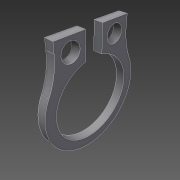
# Autodesk Inventor part: Horseshoe Clip
Saved by Autodesk Inventor 2016 (Build 200138000, 138)
## iProperties
Created: 2012-08-29
Part Number: Horseshoe Clip
Material: Generic
Document SubType Name: Modeling
Designer: John
Density: 1 g/cm^3
Appearance: Default
Author: John
Autodesk Inventor part; units mm, degrees
ref_plane "YZ Plane" through (0, 0, 0) normal (1, 0, 0) x (0, 1, 0)
ref_plane "XZ Plane" through (0, 0, 0) normal (0, 1, 0) x (-1, 0, 0)
ref_plane "XY Plane" through (0, 0, 0) normal (0, 0, 1) x (1, 0, 0)
sketch "Sketch1" plane through (0, 0, 0) normal (1, 0, 0) x (0, 1, 0)
  circle A0 centre (0, 0) radius 3.683
  line L0 (4.699, 2.6924) -> (0, 2.6924)
  line L1 (0, 2.6924) -> (0, -2.6924)
  line L2 (0, -2.6924) -> (4.699, -2.6924)
  line L3 (4.699, -2.6924) -> (4.699, 2.6924)
  dimension "d0" = 7.366
  dimension "d1" = 5.3848
  dimension "d2" = 4.699
  constraints: 8 end point, 2 coincident, 2 parallel, 1 centre point, 1 horizontal, 1 midpoint, 1 perpendicular
  measures "d0" diameter of A0
  measures "d1" distance of L2.end L0.start
  measures "d2" distance of L0.start L0.end
extrude "Extrusion1" add sketch "Sketch1" along normal blind 0.635
fillet "Fillet1" radius 5.08 2 edges at (0.3175, 2.5131, -2.6924) (0.3175, 2.5131, 2.6924)
sketch "Sketch2" plane through (0.635, 0, 0) normal (1, 0, 0) x (0, 0, -1)
  arc A0 (-3.2667, 1.701) -> (3.2667, 1.701) centre (0, 0) ccw projected
  line L0 (2.6924, 4.699) -> (-2.6924, 4.699) projected
  circle A1 centre (0, 0) radius 2.921
  line L1 (-0.635, 2.8511) -> (0.635, 2.8511)
  line L2 (0.635, 2.8511) -> (0.635, 4.699)
  line L3 (0.635, 4.699) -> (-0.635, 4.699)
  line L4 (-0.635, 4.699) -> (-0.635, 2.8511)
  dimension "d6" = 5.842
  dimension "d7" = 1.27
  constraints: 8 end point, 2 parallel, 2 point on circle, 1 centre point, 1 coincident, 1 collinear, 1 horizontal, 1 perpendicular
  measures "d6" diameter of A1
  measures "d7" distance of L2.end L3.end
extrude "Extrusion2" cut sketch "Sketch2" against normal through all
sketch "Sketch3" plane through (0.635, 0, 0) normal (1, 0, 0) x (0, 0, -1)
  line L0 (-0.635, 2.8511) -> (-2.6924, 4.699) construction
  line L1 (0.635, 2.8511) -> (2.6924, 4.699) construction
  point P0 (-1.6637, 3.7751)
  point P1 (1.6637, 3.7751)
  constraints: 4 end point, 2 midpoint
hole "Hole1" at (0.635, 3.7751, 1.6637) at (0.635, 3.7751, -1.6637) direction (-1, 0, 0) diameter 1.27 end through all
body "Solid1"
